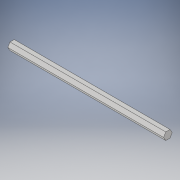
# Autodesk Inventor part: 10.5 in Hex Shaft Top Roller Wheel
Saved by Autodesk Inventor 2018 (Build 220112000, 112)
## iProperties
Created: 2020-02-25
Part Number: 10.5 in Hex Shaft Top Roller Wheel
Material: Generic
Document SubType Name: Modeling
Designer: T3500STATIC
Density: 1 g/cm^3
Appearance: Default
Author: T3500STATIC
Autodesk Inventor part; units mm, degrees
ref_plane "YZ Plane" through (0, 0, 0) normal (1, 0, 0) x (0, 1, 0)
ref_plane "XZ Plane" through (0, 0, 0) normal (0, 1, 0) x (-1, 0, 0)
ref_plane "XY Plane" through (0, 0, 0) normal (0, 0, 1) x (1, 0, 0)
sketch "Sketch1" plane through (0, 0, 0) normal (1, 0, 0) x (0, 1, 0)
  line L0 (0, 0) -> (6.35, 0) construction
  line L1 (6.35, -3.6662) -> (0, -7.3323)
  line L2 (0, -7.3323) -> (-6.35, -3.6662)
  line L3 (-6.35, -3.6662) -> (-6.35, 3.6662)
  line L4 (-6.35, 3.6662) -> (0, 7.3323)
  line L5 (0, 7.3323) -> (6.35, 3.6662)
  line L6 (6.35, 3.6662) -> (6.35, -3.6662)
  dimension "d0" = 6.35
  constraints: 14 end point, 1 coincident, 1 horizontal, 1 midpoint, 13 other
  measures "d0" distance of L0.start L0.end
extrude "Extrusion1" add sketch "Sketch1" along normal blind 266.7
body "Solid1"
